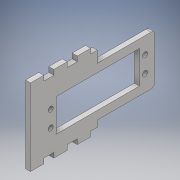
# Autodesk Inventor part: cod
Saved by Autodesk Inventor 2018 (Build 220112000, 112)
## iProperties
Created: 2020-03-11
Part Number: cod
Material: Genérico
Document SubType Name: Modeling
Designer: sala.ceri
Density: 1 g/cm^3
Appearance: Valor por defecto
Author: sala.ceri
Autodesk Inventor part; units mm, degrees
ref_plane "YZ Plane" through (0, 0, 0) normal (1, 0, 0) x (0, 1, 0)
ref_plane "XZ Plane" through (0, 0, 0) normal (0, 1, 0) x (-1, 0, 0)
ref_plane "XY Plane" through (0, 0, 0) normal (0, 0, 1) x (1, 0, 0)
sketch "Boceto1" plane through (0, 0, 0) normal (1, 0, 0) x (0, 1, 0)
  line L0 (0, 0) -> (0, -3)
  line L1 (0, -3) -> (10, -3)
  line L2 (10, -3) -> (10, 0)
  line L3 (10, 0) -> (20, 0)
  line L4 (20, 0) -> (20, -3)
  line L5 (20, -3) -> (30, -3)
  line L6 (30, -33.4269) -> (30, -40)
  line L7 (30, -40) -> (20, -40)
  line L8 (20, -40) -> (20, -43)
  line L9 (20, -43) -> (10, -43)
  line L10 (10, -43) -> (10, -40)
  line L11 (10, -40) -> (0, -40)
  circle A0 centre (15, -21.5) radius 13.175
  arc A1 (0, -9.5731) -> (0, -33.4269) centre (15, -21.5) ccw
  arc A2 (30, -33.4269) -> (30, -9.5731) centre (15, -21.5) ccw
  line L12 (0, -40) -> (0, -33.4269)
  line L13 (0, -9.5731) -> (0, -3)
  line L14 (30, -3) -> (30, -9.5731)
  dimension "d1" = 10
  dimension "d2" = 10
  dimension "d3" = 10
  constraints: 30 end point, 9 perpendicular, 9 point on line, 4 point on circle, 3 centre point, 2 parallel, 1 coincident, 1 vertical
  measures "d1" distance of L0.end L1.end
  measures "d2" distance of L2.end L3.end
  measures "d3" distance of L4.end L5.end
extrude "Extrusión1" add sketch "Boceto1" along normal blind 3
sketch "Boceto2" plane through (3, 0, 0) normal (1, 0, 0) x (0, 0, -1)
  line L0 (3, 10) -> (3, 0) projected
  line L1 (3, 0) -> (0, 0)
  line L2 (0, 20) -> (0, 10) projected
  line L3 (0, 0) -> (0, 10)
  line L4 (0, 10) -> (-3, 10)
  line L5 (-3, 10) -> (-3, 20)
  line L6 (-3, 20) -> (0, 20)
  line L7 (0, 20) -> (0, 30)
  line L8 (3, 30) -> (3, 20) projected
  line L9 (0, 30) -> (3, 30)
  line L10 (3, 30) -> (3, 20)
  line L11 (3, 20) -> (0, 20) projected
  line L12 (3, 20) -> (0, 20)
  line L13 (0, 20) -> (0, 10)
  line L14 (0, 10) -> (3, 10)
  line L15 (3, 0) -> (3, 10)
  dimension "d11" = 3
  constraints: 24 end point, 7 perpendicular, 3 point on line, 2 collinear, 1 horizontal
  measures "d11" distance of L2.end L4.end
extrude "Extrusión2" add sketch "Boceto2" against normal blind 3
sketch "Boceto3" plane through (3, 0, 0) normal (1, 0, 0) x (0, 0, -1)
  line L0 (0, 30) -> (9.5731, 30) projected
  line L1 (0, 30) -> (9.5731, 30)
  line L2 (40, 30) -> (33.4269, 30) projected
  line L3 (9.5731, 30) -> (40, 30)
  line L4 (40, 10) -> (40, 0) projected
  line L5 (40, 30) -> (40, 0)
  line L6 (9.5731, 0) -> (0, 0) projected
  line L7 (40, 0) -> (0, 0)
  line L8 (0, 30) -> (0, 20) projected
  line L9 (0, 0) -> (0, 30)
  circle A0 centre (21.5, 15) radius 26.2155
  constraints: 10 end point, 5 collinear, 1 coincident, 3 other
extrude "Extrusión3" cut sketch "Boceto3" against normal blind 10 contours A0 L6 L7 L4 L5 L2 L3 L0 | L8 L9 A0
sketch "Boceto4" plane through (3, 0, 0) normal (1, 0, 0) x (0, 0, -1)
  circle A0 centre (21.5, 15) radius 13.175 projected
  circle A1 centre (21.5, 15) radius 13.175
  circle A2 centre (21.5, 15) radius 3
  point P0 (0, 0)
  constraints: 2 centre point, 2 coincident
extrude "Extrusión4" add sketch "Boceto4" against normal blind 3
sketch "Boceto5" plane through (3, 0, 0) normal (1, 0, 0) x (0, 0, -1)
  line L0 (0, 25.951) -> (-3, 25.951)
  line L1 (-3, 25.951) -> (-3, 17.951)
  line L2 (-3, 17.951) -> (0, 17.951)
  line L3 (0, 25.951) -> (0, 17.951)
  line L4 (-3, 11.951) -> (0, 11.951)
  line L5 (0, 11.951) -> (0, 3.951)
  line L6 (0, 3.951) -> (-3, 3.951)
  line L7 (-3, 3.951) -> (-3, 11.951)
  line L8 (40, 0) -> (0, 0) projected
  line L9 (0, 0) -> (40, 0)
  line L10 (40, 25.951) -> (43, 25.951)
  line L11 (43, 25.951) -> (43, 17.951)
  line L12 (43, 17.951) -> (40, 17.951)
  line L13 (40, 25.951) -> (40, 17.951)
  line L14 (43, 11.951) -> (40, 11.951)
  line L15 (40, 11.951) -> (40, 3.951)
  line L16 (40, 3.951) -> (43, 3.951)
  line L17 (43, 3.951) -> (43, 11.951)
  constraints: 34 end point, 5 perpendicular, 1 horizontal
extrude "Extrusión5" add sketch "Boceto5" against normal blind 3
sketch "Boceto6" plane through (3, 0, 0) normal (1, 0, 0) x (0, 0, -1)
  line L0 (31.25, 30) -> (31.25, 55.25)
  line L1 (31.25, 55.25) -> (11.75, 55.25)
  line L2 (11.75, 55.25) -> (11.75, 30)
  line L3 (11.75, 60.25) -> (6.75, 60.25)
  line L4 (31.25, 60.25) -> (36.25, 60.25)
  line L5 (36.25, 60.25) -> (36.25, 30)
  line L6 (31.25, 30) -> (36.25, 30)
  line L7 (31.25, 60.25) -> (11.75, 60.25)
  line L8 (6.75, 60.25) -> (6.75, 30)
  line L9 (6.75, 30) -> (11.75, 30)
  point P0 (0, 0)
  point P1 (21.5, 15)
  constraints: 20 end point, 2 perpendicular, 2 vertical, 1 horizontal
extrude "Extrusión6" add sketch "Boceto6" against normal blind 3
sketch "Boceto7" plane through (3, 0, 0) normal (1, 0, 0) x (0, 0, -1)
  line L0 (11.75, 30.1448) -> (11.75, 5.25)
  line L1 (11.75, 5.25) -> (31.25, 5.25)
  line L2 (31.25, 5.25) -> (31.25, 30.1448)
  line L3 (31.25, 30.1448) -> (11.75, 30.1448)
  point P0 (0, 0)
  point P1 (21.5, 15)
  constraints: 8 end point, 3 perpendicular, 1 vertical
extrude "Extrusión7" cut sketch "Boceto7" against normal blind 3
sketch "Boceto8" plane through (3, 0, 0) normal (1, 0, 0) x (0, 0, -1)
  line L0 (0, -2.049) -> (-3, -2.049)
  line L1 (-3, -2.049) -> (-3, -10.049)
  line L2 (40, 0) -> (40, -2.049)
  line L3 (40, -2.049) -> (43, -2.049)
  line L4 (43, -2.049) -> (43, -10.049)
  line L5 (43, -10.049) -> (-3, -10.049)
  line L6 (0, 0) -> (0, -2.049)
  line L7 (6.75, 60.25) -> (6.75, 64.25)
  line L8 (36.25, 60.25) -> (36.25, 64.25)
  line L9 (36.25, 64.25) -> (6.75, 64.25)
  line L10 (6.75, 60.25) -> (36.25, 60.25) projected
  line L11 (6.75, 60.25) -> (36.25, 60.25)
  line L12 (40, 0) -> (0, 0) projected
  line L13 (0, 0) -> (40, 0)
  point P0 (0, 3.951)
  dimension "d50" = 4
  constraints: 24 end point, 5 perpendicular, 4 vertical, 1 collinear, 1 horizontal
  measures "d50" distance of L7.start L7.end
extrude "Extrusión8" add sketch "Boceto8" against normal blind 3
sketch "Boceto9" plane through (3, 0, 0) normal (1, 0, 0) x (0, 0, -1)
  circle A0 centre (26.375, 58.5) radius 1.5
  circle A1 centre (16.625, 58.5) radius 1.5
  circle A2 centre (26.375, 2) radius 1.5
  circle A3 centre (16.625, 2) radius 1.5
  point P0 (0, 0)
  constraints: 4 centre point
extrude "Extrusión9" cut sketch "Boceto9" against normal blind 3
fillet "Empalme1" radius 2 2 edges at (1.5, 64.25, -6.75) (1.5, 64.25, -36.25)
